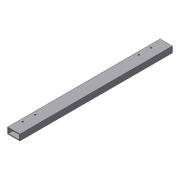
# Autodesk Inventor part: Frame_SideRail_Inner_2x1
Saved by Autodesk Inventor 2012 (Build 160160000, 160)
## iProperties
Created: 2012-01-08
Part Number: Frame_SideRail_Inner_2x1
Material: Aluminum-6061
Document SubType Name: Modeling
Designer: JesseK
Mass: 761.099 g
Surface Area: 1783.06 cm^2
Volume: 280.848 cm^3
Density: 2.71 g/cm^3
Author: JesseK
Autodesk Inventor part; units mm, degrees
ref_plane "YZ Plane" through (0, 0, 0) normal (1, 0, 0) x (0, 1, 0)
ref_plane "XZ Plane" through (0, 0, 0) normal (0, 1, 0) x (-1, 0, 0)
ref_plane "XY Plane" through (0, 0, 0) normal (0, 0, 1) x (1, 0, 0)
sketch "Sketch1" plane through (0, 0, 0) normal (0, 0, 1) x (1, 0, 0)
  line L0 (0, 0) -> (50.8, 0)
  line L1 (50.8, 0) -> (50.8, 25.4)
  line L2 (50.8, 25.4) -> (0, 25.4)
  line L3 (0, 25.4) -> (0, 0)
  dimension "d0" = 25.4
  dimension "d1" = 50.8
  constraints: 8 end point, 2 parallel, 1 horizontal, 1 perpendicular
  measures "d0" distance of L2.end L0.start
  measures "d1" distance of L0.start L0.end
extrude "Extrusion1" add sketch "Sketch1" along normal blind 635
shell "Shell1" thickness 3.175 removed faces 2 at (16.9333, 16.9333, 0) at (33.8667, 8.4667, 635)
sketch "Sketch2" plane through (0, 25.4, 0) normal (0, 1, 0) x (1, 0, 0)
  line L0 (0, -635) -> (50.8, -635) projected
  line L1 (50.8, 0) -> (0, 0) projected
  line L2 (0, 0) -> (0, -635) projected
  line L3 (12.7, 0) -> (12.7, -50.8) construction
  line L4 (12.7, -50.8) -> (12.7, -101.6) construction
  line L5 (12.7, -101.6) -> (12.7, -533.4) construction
  line L6 (12.7, -533.4) -> (12.7, -584.2) construction
  line L7 (12.7, -584.2) -> (12.7, -635) construction
  circle A0 centre (12.7, -50.8) radius 3.175
  circle A1 centre (12.7, -101.6) radius 3.175
  circle A2 centre (12.7, -533.4) radius 3.175
  circle A3 centre (12.7, -584.2) radius 3.175
  dimension "d4" = 12.7
  dimension "d5" = 50.8
  dimension "d6" = 50.8
  dimension "d7" = 6.35
  dimension "d8" = 6.35
  dimension "d9" = 6.35
  dimension "d10" = 6.35
  constraints: 10 end point, 4 centre point, 4 coincident, 3 collinear, 3 parallel, 2 point on line, 1 perpendicular
  measures "d4" distance between parallel lines of L2 L5
  measures "d5" distance of L3.end L4.end
  measures "d6" distance of L3.start L3.end
  measures "d7" diameter of A2
  measures "d8" diameter of A3
  measures "d9" diameter of A0
  measures "d10" diameter of A1
extrude "Extrusion2" cut sketch "Sketch2" against normal through all
body "Solid1"
